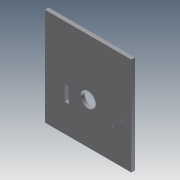
# Autodesk Inventor part: frontbase
Saved by Autodesk Inventor 2011 (Build 150239000, 239)
## iProperties
Created: 2011-12-11
Part Number: frontbase
Document SubType Name: Modeling
Designer: Matthew
Density: 1 g/cm^3
Author: Matthew
Autodesk Inventor part; units mm, degrees
ref_plane "YZ Plane" through (0, 0, 0) normal (1, 0, 0) x (0, 1, 0)
ref_plane "XZ Plane" through (0, 0, 0) normal (0, 1, 0) x (-1, 0, 0)
ref_plane "XY Plane" through (0, 0, 0) normal (0, 0, 1) x (1, 0, 0)
sketch "Sketch1" plane through (0, 0, 0) normal (0, 0, 1) x (1, 0, 0)
  line L0 (-19.7465, 14.2682) -> (107.2535, 14.2682)
  line L1 (107.2535, 14.2682) -> (107.2535, -112.7318)
  line L2 (107.2535, -112.7318) -> (-19.7465, -112.7318)
  line L3 (-19.7465, -112.7318) -> (-19.7465, 14.2682)
  point P0 (0, 0)
  dimension "d0" = 127
  dimension "d1" = 127
  constraints: 8 end point, 2 parallel, 1 horizontal, 1 perpendicular
  measures "d0" distance of L1.end L2.end
  measures "d1" distance of L0.end L1.end
extrude "Extrusion1" add sketch "Sketch1" along normal blind 6.35
sketch "Sketch2" plane through (0, 0, 6.35) normal (0, 0, 1) x (1, 0, 0)
  line L0 (107.2535, -112.7318) -> (-19.7465, -112.7318) projected
  line L1 (-19.7465, -112.7318) -> (43.7535, -112.7318)
  line L2 (43.7535, -112.7318) -> (43.7535, -61.9318)
  line L3 (43.7535, -61.9318) -> (66.7535, -61.9318)
  line L4 (66.7535, -61.9318) -> (73.1035, -61.9318)
  line L5 (73.1035, -61.9318) -> (113.1035, -61.9318)
  line L6 (113.1035, -61.9318) -> (113.1035, -93.9318)
  line L7 (113.1035, -93.9318) -> (73.1035, -93.9318)
  line L8 (73.1035, -93.9318) -> (73.1035, -61.9318)
  point P0 (0, 0)
  dimension "d4" = 50.8
  dimension "d5" = 23
  dimension "d6" = 6.35
  dimension "d7" = 40
  dimension "d8" = 32
  constraints: 16 end point, 3 perpendicular, 2 parallel, 1 collinear, 1 horizontal, 1 midpoint
  measures "d4" distance of L1.end L2.end
  measures "d5" distance of L2.end L3.end
  measures "d6" distance of L3.end L4.end
  measures "d7" distance of L6.end L7.end
  measures "d8" distance of L5.end L6.end
extrude "Extrusion2" add sketch "Sketch2" along normal blind 6.35
sketch "Sketch3" plane through (107.2535, -112.7318, 0) normal (1, 0, 0) x (0, 0, -1)
  line L0 (-6.35, 127) -> (-6.35, 50.8) projected
  line L1 (-6.35, 50.8) -> (-6.35, 18.8) projected
  line L2 (-6.35, 18.8) -> (-6.35, 0) projected
  line L3 (0, 0) -> (-6.35, 0) projected
  line L4 (0, 127) -> (0, 0) projected
  line L5 (0, 127) -> (-6.35, 127) projected
  point P0 (0, 112.7318)
extrude "Extrusion3" add sketch "Sketch3" along normal blind 12.7
sketch "Sketch4" plane through (-19.7465, -112.7318, 0) normal (-1, 0, 0) x (0, 0, 1)
  line L0 (6.35, 0) -> (6.35, 127) projected
  line L1 (0, 127) -> (6.35, 127) projected
  line L2 (0, 0) -> (0, 127) projected
  line L3 (0, 0) -> (6.35, 0) projected
  point P0 (0, 112.7318)
extrude "Extrusion4" add sketch "Sketch4" along normal blind 12.7
sketch "Sketch5" plane through (0, 0, 6.35) normal (0, 0, 1) x (1, 0, 0)
  line L0 (119.9535, -112.7318) -> (-32.4465, -112.7318) projected
  line L1 (119.9535, -112.7318) -> (43.7535, -112.7318)
  line L2 (43.7535, -112.7318) -> (43.7535, -61.9318)
  line L3 (43.7535, -61.9318) -> (20.7535, -61.9318)
  line L4 (20.7535, -61.9318) -> (14.4035, -61.9318)
  line L5 (14.4035, -61.9318) -> (8.0535, -61.9318)
  line L6 (8.0535, -61.9318) -> (14.4035, -61.9318)
  line L7 (14.4035, -61.9318) -> (14.4035, -87.3318)
  line L8 (14.4035, -87.3318) -> (8.0535, -87.3318)
  line L9 (8.0535, -87.3318) -> (8.0535, -61.9318)
  point P0 (0, 0)
  dimension "d15" = 23
  dimension "d16" = 6.35
  dimension "d17" = 6.35
  dimension "d18" = 25.4
  constraints: 18 end point, 3 perpendicular, 2 collinear, 2 parallel, 1 horizontal, 1 midpoint
  measures "d15" distance of L2.end L3.end
  measures "d16" distance of L3.end L4.end
  measures "d17" distance of L4.end L5.end
  measures "d18" distance of L6.end L7.end
extrude "Extrusion5" cut sketch "Sketch5" against normal blind 12.7
sketch "Sketch6" plane through (0, 0, 6.35) normal (0, 0, 1) x (1, 0, 0)
  line L0 (119.9535, -112.7318) -> (119.9535, 14.2682) projected
  line L1 (113.1035, -61.9318) -> (119.9535, -61.9318)
  line L2 (119.9535, -61.9318) -> (119.9535, -93.9318)
  line L3 (119.9535, -93.9318) -> (113.1035, -93.9318)
  line L4 (113.1035, -93.9318) -> (113.1035, -61.9318)
  point P0 (0, 0)
  constraints: 8 end point, 2 parallel, 1 horizontal, 1 perpendicular, 1 point on line
extrude "Extrusion6" cut sketch "Sketch6" against normal blind 12.7
sketch "Sketch7" plane through (0, 0, 12.7) normal (0, 0, 1) x (1, 0, 0)
  line L0 (73.1035, -61.9318) -> (113.1035, -61.9318) projected
  line L1 (73.1035, -93.9318) -> (73.1035, -61.9318) projected
  line L2 (113.1035, -93.9318) -> (73.1035, -93.9318) projected
  line L3 (113.1035, -61.9318) -> (113.1035, -93.9318) projected
  point P0 (0, 0)
extrude "Extrusion7" cut sketch "Sketch7" against normal blind 6.35
sketch "Sketch8" plane through (0, 0, 6.35) normal (0, 0, 1) x (1, 0, 0)
  line L0 (14.4035, -61.9318) -> (14.4035, -87.3318) projected
  line L1 (113.1035, -61.9318) -> (4.4035, -61.9318)
  line L2 (4.4035, -61.9318) -> (8.0535, -61.9318)
  line L3 (8.0535, -61.9318) -> (8.0535, -87.3318)
  line L4 (8.0535, -87.3318) -> (4.4035, -87.3318)
  line L5 (4.4035, -87.3318) -> (4.4035, -61.9318)
  point P0 (0, 0)
  dimension "d25" = 108.7
  constraints: 10 end point, 2 parallel, 2 perpendicular, 1 horizontal
  measures "d25" distance of L1.start L1.end
extrude "Extrusion8" cut sketch "Sketch8" against normal blind 6.35
sketch "Sketch9" plane through (0, 0, 6.35) normal (0, 0, 1) x (1, 0, 0)
  line L0 (4.4035, -61.9318) -> (14.4035, -61.9318) projected
  line L1 (14.4035, -61.9318) -> (14.4035, -87.3318) projected
  line L2 (14.4035, -87.3318) -> (4.4035, -87.3318) projected
  line L3 (4.4035, -87.3318) -> (4.4035, -61.9318) projected
  line L4 (4.4035, -61.9318) -> (10.7535, -61.9318)
  line L5 (10.7535, -61.9318) -> (10.7535, -87.3318)
  line L6 (10.7535, -87.3318) -> (4.4035, -87.3318)
  line L7 (4.4035, -87.3318) -> (4.4035, -61.9318)
  point P0 (0, 0)
  dimension "d28" = 6.35
  constraints: 8 end point, 2 parallel, 1 horizontal, 1 perpendicular, 1 point on line
  measures "d28" distance of L5.end L6.end
extrude "Extrusion9" add sketch "Sketch9" against normal blind 6.35 contours L0 L1 L2 L5
sketch "Sketch10" plane through (0, 0, 0) normal (0, 0, -1) x (-1, 0, 0)
  line L0 (-113.1035, -61.9318) -> (-101.1035, -61.9318)
  line L1 (-101.1035, -61.9318) -> (-101.1035, -69.9318)
  line L2 (-101.1035, -69.9318) -> (-113.1035, -69.9318)
  line L3 (-113.1035, -69.9318) -> (-113.1035, -61.9318)
  line L4 (-101.1035, -69.9318) -> (-85.1035, -69.9318)
  line L5 (-85.1035, -69.9318) -> (-85.1035, -85.9318)
  line L6 (-85.1035, -85.9318) -> (-101.1035, -85.9318)
  line L7 (-101.1035, -85.9318) -> (-101.1035, -69.9318)
  circle A0 centre (-101.1035, -69.9318) radius 1
  circle A1 centre (-85.1035, -85.9318) radius 1
  point P0 (0, 0)
  dimension "d31" = 12
  dimension "d32" = 8
  dimension "d33" = 16
  dimension "d34" = 16
  dimension "d35" = 2
  dimension "d36" = 2
  constraints: 16 end point, 4 parallel, 2 centre point, 2 coincident, 2 horizontal, 2 perpendicular
  measures "d31" distance of L1.end L2.end
  measures "d32" distance of L0.end L1.end
  measures "d33" distance of L5.end L6.end
  measures "d34" distance of L4.end L5.end
  measures "d35" diameter of A0
  measures "d36" diameter of A1
extrude "Extrusion10" cut sketch "Sketch10" against normal blind 6.35 contours A0 L4 L1 | L1 L2 A0 | L2 L7 A0 | L4 A0 L7 | A1 L6 L5 | L5 L6 A1
sketch "Sketch11" plane through (113.1035, -93.9318, 6.35) normal (1, 0, 0) x (0, 0, -1)
  line L0 (0, 32) -> (0, 0) projected
  line L1 (0, 0) -> (6.35, 0) projected
  line L2 (6.35, 32) -> (6.35, 0) projected
  line L3 (0, 32) -> (6.35, 32) projected
  point P0 (6.35, 93.9318)
extrude "Extrusion11" add sketch "Sketch11" along normal blind 7.62
sketch "Sketch12" plane through (119.9535, -112.7318, 0) normal (1, 0, 0) x (0, 0, -1)
  line L0 (-6.35, 50.8) -> (0, 50.8)
  line L1 (0, 50.8) -> (0, 11.311)
  line L2 (0, 11.311) -> (-6.35, 11.311)
  line L3 (-6.35, 11.311) -> (-6.35, 50.8)
  point P0 (0, 112.7318)
  constraints: 8 end point, 2 parallel, 1 horizontal, 1 perpendicular
extrude "Extrusion12" cut sketch "Sketch12" along normal blind 7.62
sketch "Sketch13" plane through (0, 0, 0) normal (0, 0, -1) x (-1, 0, 0)
  line L0 (-10.7535, -87.3318) -> (-4.4035, -87.3318)
  line L1 (-4.4035, -87.3318) -> (-4.4035, -90.6318)
  line L2 (-4.4035, -90.6318) -> (-10.7535, -90.6318)
  line L3 (-10.7535, -90.6318) -> (-10.7535, -87.3318)
  point P0 (0, 0)
  dimension "d43" = 3.3
  constraints: 8 end point, 2 parallel, 1 horizontal, 1 perpendicular
  measures "d43" distance of L0.end L1.end
extrude "Extrusion13" cut sketch "Sketch13" against normal blind 7.62
sketch "Sketch14" plane through (0, 0, 0) normal (0, 0, -1) x (-1, 0, 0)
  line L0 (-4.4035, -61.9318) -> (-4.4035, -90.6318) projected
  line L1 (-10.7535, -61.9318) -> (-4.4035, -61.9318)
  line L2 (-4.4035, -61.9318) -> (-4.4035, -65.2318)
  line L3 (-4.4035, -65.2318) -> (-10.7535, -65.2318)
  line L4 (-10.7535, -65.2318) -> (-10.7535, -61.9318)
  point P0 (0, 0)
  dimension "d46" = 3.3
  constraints: 8 end point, 2 parallel, 1 horizontal, 1 perpendicular, 1 point on line
  measures "d46" distance of L1.end L2.end
extrude "Extrusion14" add sketch "Sketch14" against normal blind 7.62
sketch "Sketch15" plane through (0, 0, 7.62) normal (0, 0, 1) x (1, 0, 0)
  line L0 (10.7535, -65.2318) -> (4.4035, -65.2318) projected
  line L1 (10.7535, -61.9318) -> (10.7535, -65.2318) projected
  line L2 (4.4035, -61.9318) -> (10.7535, -61.9318) projected
  line L3 (4.4035, -65.2318) -> (4.4035, -61.9318) projected
  point P0 (0, 0)
extrude "Extrusion15" cut sketch "Sketch15" against normal blind 1.27
sketch "Sketch16" plane through (119.9535, -112.7318, 0) normal (0, -1, 0) x (1, 0, 0)
  line L0 (0, 6.35) -> (-152.4, 6.35) projected
  line L1 (-152.4, 6.35) -> (-152.4, 0) projected
  line L2 (0, 0) -> (-152.4, 0) projected
  line L3 (0, 0) -> (0, 6.35) projected
  point P0 (-119.9535, 0)
extrude "Extrusion16" add sketch "Sketch16" along normal blind 25.4
sketch "Sketch17" plane through (119.9535, 14.2682, 6.35) normal (0, 1, 0) x (1, 0, 0)
  line L0 (-152.4, 0) -> (0, 0) projected
  line L1 (-152.4, 6.35) -> (0, 6.35) projected
  line L2 (0, 0) -> (-6.35, 0)
  line L3 (-6.35, 0) -> (-6.35, 6.35)
  line L4 (-6.35, 6.35) -> (0, 6.35)
  line L5 (0, 6.35) -> (0, 0)
  line L6 (-152.4, 6.35) -> (-146.05, 6.35)
  line L7 (-146.05, 6.35) -> (-146.05, 0)
  line L8 (-146.05, 0) -> (-152.4, 0)
  line L9 (-152.4, 0) -> (-152.4, 6.35)
  point P0 (-119.9535, 6.35)
  dimension "d53" = 6.35
  dimension "d54" = 6.35
  constraints: 16 end point, 4 parallel, 2 horizontal, 2 perpendicular, 2 point on line
  measures "d53" distance of L3.end L4.end
  measures "d54" distance of L7.end L8.end
extrude "Extrusion17" cut sketch "Sketch17" against normal blind 177.8 contours L9 L1 L7 L0 | L3 L1 L5 L0
sketch "Sketch18" plane through (0, 0, 0) normal (0, 0, -1) x (-1, 0, 0)
  line L0 (-113.6035, -138.1318) -> (26.0965, -138.1318) projected
  line L1 (-10.7535, -65.2318) -> (-4.4035, -65.2318) projected
  line L2 (-43.7535, -138.1318) -> (-43.7535, -112.7318)
  circle A0 centre (-43.7535, -112.7318) radius 12.7
  point P0 (0, 0)
  dimension "d57" = 25.4
  dimension "d58" = 25.4
  constraints: 2 end point, 1 centre point, 1 coincident, 1 midpoint, 1 perpendicular
  measures "d57" distance of L2.start L2.end
  measures "d58" diameter of A0
extrude "Extrusion18" cut sketch "Sketch18" against normal blind 25.4
sketch "Sketch19" plane through (0, 0, 0) normal (0, 0, -1) x (-1, 0, 0)
  line L0 (-113.6035, -138.1318) -> (26.0965, -138.1318) projected
  line L1 (-10.7535, -65.2318) -> (-4.4035, -65.2318) projected
  line L2 (-43.7535, -138.1318) -> (-43.7535, -68.2818)
  circle A0 centre (-43.7535, -68.2818) radius 12.7
  point P0 (0, 0)
  dimension "d61" = 69.85
  dimension "d62" = 25.4
  constraints: 2 end point, 1 centre point, 1 coincident, 1 midpoint, 1 perpendicular
  measures "d61" distance of L2.start L2.end
  measures "d62" diameter of A0
extrude "Extrusion19" cut sketch "Sketch19" against normal blind 25.4
sketch "Sketch20" plane through (0, 0, 0) normal (0, 0, -1) x (-1, 0, 0)
  circle A0 centre (-43.7535, -112.7318) radius 12.7 projected
  point P0 (0, 0)
extrude "Extrusion20" add sketch "Sketch20" against normal blind 6.35
sketch "Sketch21" plane through (-26.0965, 14.2682, 6.35) normal (0, 1, 0) x (1, 0, 0)
  line L0 (0, 6.35) -> (0, 0) projected
  line L1 (0, 0) -> (139.7, 0) projected
  line L2 (139.7, 0) -> (139.7, 6.35) projected
  line L3 (0, 6.35) -> (139.7, 6.35) projected
  point P0 (26.0965, 6.35)
extrude "Extrusion21" add sketch "Sketch21" along normal blind 12.7
sketch "Sketch22" plane through (113.6035, -138.1318, 6.35) normal (1, 0, 0) x (0, 0, -1)
  line L0 (6.35, 0) -> (0, 0) projected
  line L1 (6.35, 165.1) -> (6.35, 0) projected
  line L2 (6.35, 165.1) -> (0, 165.1) projected
  line L3 (0, 0) -> (0, 165.1) projected
  point P0 (6.35, 138.1318)
extrude "Extrusion22" add sketch "Sketch22" along normal blind 3.175
sketch "Sketch23" plane through (-26.0965, -138.1318, 0) normal (-1, 0, 0) x (0, 0, 1)
  line L0 (6.35, 0) -> (0, 0) projected
  line L1 (6.35, 165.1) -> (6.35, 0) projected
  line L2 (6.35, 165.1) -> (0, 165.1) projected
  line L3 (0, 0) -> (0, 165.1) projected
  point P0 (0, 138.1318)
extrude "Extrusion23" add sketch "Sketch23" along normal blind 3.175
sketch "Sketch24" plane through (0, 0, 6.35) normal (0, 0, 1) x (1, 0, 0)
  line L0 (4.4035, -65.2318) -> (1.2285, -65.2318)
  line L1 (1.2285, -65.2318) -> (1.2285, -90.6318)
  line L2 (1.2285, -90.6318) -> (4.4035, -90.6318)
  line L3 (4.4035, -90.6318) -> (4.4035, -65.2318)
  point P0 (0, 0)
  dimension "d73" = 3.175
  constraints: 8 end point, 2 parallel, 1 horizontal, 1 perpendicular
  measures "d73" distance of L2.end L1.end
extrude "Extrusion24" cut sketch "Sketch24" against normal blind 6.35
sketch "Sketch25" plane through (0, 0, 6.35) normal (0, 0, 1) x (1, 0, 0)
  line L0 (10.7535, -65.2318) -> (7.5785, -65.2318)
  line L1 (7.5785, -65.2318) -> (7.5785, -91.3197)
  line L2 (7.5785, -91.3197) -> (10.7535, -91.3197)
  line L3 (10.7535, -91.3197) -> (10.7535, -65.2318)
  point P0 (0, 0)
  dimension "d76" = 3.175
  constraints: 8 end point, 2 parallel, 1 horizontal, 1 perpendicular
  measures "d76" distance of L2.end L1.end
extrude "Extrusion25" add sketch "Sketch25" against normal blind 6.35
sketch "Sketch26" plane through (0, 0, 0) normal (0, 0, -1) x (-1, 0, 0)
  circle A0 centre (-101.1035, -69.9318) radius 1 projected
  circle A1 centre (-85.1035, -85.9318) radius 1 projected
  line L0 (-1.2285, -90.6318) -> (-7.5785, -90.6318) projected
  line L1 (-101.1035, -69.9318) -> (-104.2785, -69.9318)
  line L2 (-85.1035, -85.9318) -> (-88.2785, -85.9318)
  circle A2 centre (-104.2785, -69.9318) radius 1
  circle A3 centre (-88.2785, -85.9318) radius 1
  point P0 (0, 0)
  dimension "d79" = 3.175
  dimension "d80" = 3.175
  constraints: 4 end point, 2 centre point, 2 coincident, 2 parallel
  measures "d79" distance of L1.start L1.end
  measures "d80" distance of L2.start L2.end
extrude "Extrusion26" cut sketch "Sketch26" against normal blind 6.35 contours A2 | A3
sketch "Sketch27" plane through (0, 0, 0) normal (0, 0, -1) x (-1, 0, 0)
  circle A0 centre (-101.1035, -69.9318) radius 1 projected
  circle A1 centre (-85.1035, -85.9318) radius 1 projected
  point P0 (0, 0)
extrude "Extrusion27" add sketch "Sketch27" against normal blind 6.35
body "Solid1"
